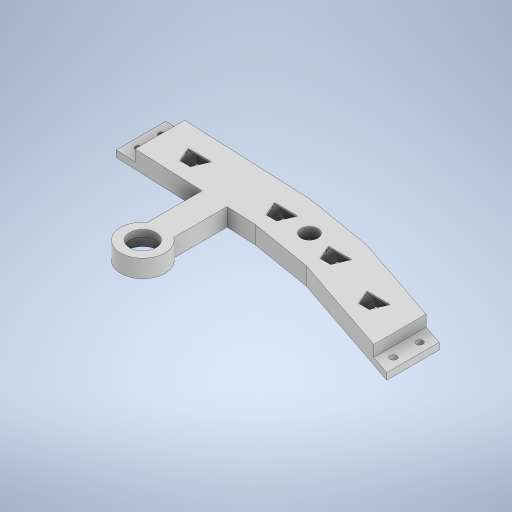
# Autodesk Inventor part: Potentiometer Holder
Saved by Autodesk Inventor 2023 (Build 270158000, 158)
## iProperties
Created: 2022-10-21
Part Number: Potentiometer Holder
Material: Generic
Document SubType Name: Modeling
Designer: GROS
Density: 1 g/cm^3
Appearance: Default
Author: GROS
Autodesk Inventor part; units mm, degrees
ref_plane "YZ Plane" through (0, 0, 0) normal (1, 0, 0) x (0, 1, 0)
ref_plane "XZ Plane" through (0, 0, 0) normal (0, 1, 0) x (-1, 0, 0)
ref_plane "XY Plane" through (0, 0, 0) normal (0, 0, 1) x (1, 0, 0)
sketch "Sketch1" plane through (0, 0, 0) normal (0, 1, 0) x (-1, 0, 0)
  line L0 (104.2041, -28.2127) -> (104.2041, -21.1501)
  line L1 (100.2041, -28.2127) -> (104.2041, -28.2127)
  line L2 (16.1749, -17.7633) -> (10.1749, -17.7633)
  line L3 (10.1749, -17.7633) -> (10.1749, -19.7955)
  line L4 (13.1749, -17.7633) -> (13.1749, -20.8106)
  line L5 (13.1749, -20.8106) -> (13.1749, -4.8696)
  line L6 (13.1749, -20.8106) -> (13.1749, -16.8106)
  line L7 (13.1749, -4.8696) -> (13.1749, -8.8696)
  circle A0 centre (13.1749, -8.8696) radius 1
  circle A1 centre (13.1749, -16.8106) radius 1
  line L8 (10.1749, -19.7955) -> (10.1749, -3.8545)
  circle A2 centre (45.4573, -23.7633) radius 7.55
  line L9 (27.7249, -17.7633) -> (20.1749, -17.7633)
  circle A3 centre (27.7249, -17.7633) radius 7.55
  line L10 (51.451, -33.7618) -> (1.5927, -16.8916)
  line L11 (20.1749, -17.7633) -> (16.1749, -17.7633)
  line L12 (16.1749, -17.7633) -> (16.1749, -5.8847)
  line L13 (16.1749, -17.7633) -> (16.1749, -21.8257)
  circle A4 centre (65.1803, -27.0368) radius 7.55
  line L14 (70.678, -35.6025) -> (39.5208, -30.4313)
  line L15 (107.2041, -28.2127) -> (107.2041, -21.2785)
  line L16 (107.2041, -21.2785) -> (107.2041, -25.2785)
  line L17 (104.2041, -28.2127) -> (104.2041, -36.2639)
  circle A5 centre (107.2041, -32.3923) radius 1
  line L18 (110.2041, -28.2127) -> (110.2041, -21.4069)
  line L19 (107.2041, -28.2127) -> (107.2041, -36.3923)
  line L20 (107.2041, -36.3923) -> (107.2041, -28.3923)
  line L21 (104.2041, -28.2127) -> (110.2041, -28.2127)
  line L22 (110.2041, -28.2127) -> (110.2041, -36.5208)
  circle A6 centre (107.2041, -25.2785) radius 1
  line L23 (114.6217, -21.596) -> (60.8612, -19.295)
  line L24 (60.2143, -34.3811) -> (122.676, -37.0546)
  line L25 (92.6541, -28.2127) -> (100.2041, -28.2127)
  circle A7 centre (92.6541, -28.2127) radius 7.55
  line L26 (51.8932, -17.9704) -> (4.2209, -1.8399)
  line L27 (75.2254, -21.0507) -> (39.3363, -15.0941)
  line L28 (55.3188, -33.0533) -> (55.3188, -17.7467)
  circle A8 centre (55.3188, -25.4) radius 2.55
  circle A9 centre (55.3188, -25.4) radius 1
  line L29 (65.1803, -27.0368) -> (45.4573, -27.0368)
  line L30 (92.6541, -35.7627) -> (92.6541, -28.2127)
  line L31 (65.1803, -34.5868) -> (65.1803, -27.0368)
  line L32 (45.4573, -31.3133) -> (45.4573, -23.7633)
  line L33 (27.7249, -25.3133) -> (27.7249, -17.7633)
  line L34 (92.6541, -28.2127) -> (92.6541, -35.7627)
  line L35 (96.1541, -28.3227) -> (95.1941, -28.3227)
  circle A10 centre (95.1941, -28.3227) radius 0.5
  line L36 (96.1541, -29.3227) -> (93.9142, -23.965)
  line L37 (90.1141, -29.3227) -> (89.1541, -29.3227)
  line L38 (90.1141, -28.3227) -> (90.1141, -29.3227)
  line L39 (89.1541, -29.3227) -> (91.4835, -23.7509)
  circle A11 centre (90.1141, -28.3227) radius 0.5
  line L40 (95.1941, -28.3227) -> (92.6541, -28.3227)
  line L41 (92.6541, -28.3227) -> (92.6541, -25.7827)
  circle A12 centre (92.6541, -25.7827) radius 0.5
  line L42 (92.6541, -28.3227) -> (90.1141, -28.3227)
  line L43 (96.1541, -32.0527) -> (96.1541, -24.8527)
  line L44 (96.1541, -32.0527) -> (96.1541, -28.3227)
  line L45 (96.1541, -24.8527) -> (89.1541, -24.8527)
  line L46 (89.1541, -24.8527) -> (89.1541, -32.0527)
  line L47 (92.6541, -32.0527) -> (96.1541, -32.0527)
  line L48 (89.1541, -29.3227) -> (96.1541, -29.3227)
  line L49 (89.1541, -32.0527) -> (96.1541, -32.0527)
  line L50 (92.6541, -28.2127) -> (92.6541, -32.0527)
  line L51 (92.6541, -35.7627) -> (92.6541, -28.2127)
  line L52 (65.1803, -27.0368) -> (65.1803, -34.5868)
  line L53 (68.6803, -27.1468) -> (67.7203, -27.1468)
  circle A13 centre (67.7203, -27.1468) radius 0.5
  line L54 (68.6803, -28.1468) -> (66.4404, -22.789)
  line L55 (62.6403, -28.1468) -> (61.6803, -28.1468)
  line L56 (62.6403, -27.1468) -> (62.6403, -28.1468)
  line L57 (61.6803, -28.1468) -> (64.0097, -22.5749)
  circle A14 centre (62.6403, -27.1468) radius 0.5
  line L58 (67.7203, -27.1468) -> (65.1803, -27.1468)
  line L59 (65.1803, -27.1468) -> (65.1803, -24.6068)
  circle A15 centre (65.1803, -24.6068) radius 0.5
  line L60 (65.1803, -27.1468) -> (62.6403, -27.1468)
  line L61 (68.6803, -30.8768) -> (68.6803, -23.6768)
  line L62 (68.6803, -30.8768) -> (68.6803, -27.1468)
  line L63 (68.6803, -23.6768) -> (61.6803, -23.6768)
  line L64 (61.6803, -23.6768) -> (61.6803, -30.8768)
  line L65 (65.1803, -30.8768) -> (68.6803, -30.8768)
  line L66 (61.6803, -28.1468) -> (68.6803, -28.1468)
  line L67 (61.6803, -30.8768) -> (68.6803, -30.8768)
  line L68 (65.1803, -27.0368) -> (65.1803, -30.8768)
  line L69 (65.1803, -34.5868) -> (65.1803, -27.0368)
  line L70 (45.4573, -23.7633) -> (45.4573, -31.3133)
  line L71 (48.9573, -23.8733) -> (47.9973, -23.8733)
  circle A16 centre (47.9973, -23.8733) radius 0.5
  line L72 (48.9573, -24.8733) -> (46.7174, -19.5156)
  line L73 (42.9173, -24.8733) -> (41.9573, -24.8733)
  line L74 (42.9173, -23.8733) -> (42.9173, -24.8733)
  line L75 (41.9573, -24.8733) -> (44.2867, -19.3014)
  circle A17 centre (42.9173, -23.8733) radius 0.5
  line L76 (47.9973, -23.8733) -> (45.4573, -23.8733)
  line L77 (45.4573, -23.8733) -> (45.4573, -21.3333)
  circle A18 centre (45.4573, -21.3333) radius 0.5
  line L78 (45.4573, -23.8733) -> (42.9173, -23.8733)
  line L79 (48.9573, -27.6033) -> (48.9573, -20.4033)
  line L80 (48.9573, -27.6033) -> (48.9573, -23.8733)
  line L81 (48.9573, -20.4033) -> (41.9573, -20.4033)
  line L82 (41.9573, -20.4033) -> (41.9573, -27.6033)
  line L83 (45.4573, -27.6033) -> (48.9573, -27.6033)
  line L84 (41.9573, -24.8733) -> (48.9573, -24.8733)
  line L85 (41.9573, -27.6033) -> (48.9573, -27.6033)
  line L86 (45.4573, -23.7633) -> (45.4573, -27.6033)
  line L87 (45.4573, -31.3133) -> (45.4573, -23.7633)
  line L88 (27.7249, -17.7633) -> (27.7249, -25.3133)
  line L89 (31.2249, -17.8733) -> (30.2649, -17.8733)
  circle A19 centre (30.2649, -17.8733) radius 0.5
  line L90 (31.2249, -18.8733) -> (28.985, -13.5156)
  line L91 (25.1849, -18.8733) -> (24.2249, -18.8733)
  line L92 (25.1849, -17.8733) -> (25.1849, -18.8733)
  line L93 (24.2249, -18.8733) -> (26.5542, -13.3014)
  circle A20 centre (25.1849, -17.8733) radius 0.5
  line L94 (30.2649, -17.8733) -> (27.7249, -17.8733)
  line L95 (27.7249, -17.8733) -> (27.7249, -15.3333)
  circle A21 centre (27.7249, -15.3333) radius 0.5
  line L96 (27.7249, -17.8733) -> (25.1849, -17.8733)
  line L97 (31.2249, -21.6033) -> (31.2249, -14.4033)
  line L98 (31.2249, -21.6033) -> (31.2249, -17.8733)
  line L99 (31.2249, -14.4033) -> (24.2249, -14.4033)
  line L100 (24.2249, -14.4033) -> (24.2249, -21.6033)
  line L101 (27.7249, -21.6033) -> (31.2249, -21.6033)
  line L102 (24.2249, -18.8733) -> (31.2249, -18.8733)
  line L103 (24.2249, -21.6033) -> (31.2249, -21.6033)
  line L104 (27.7249, -17.7633) -> (27.7249, -21.6033)
  line L105 (27.7249, -25.3133) -> (27.7249, -17.7633)
  line L106 (92.6541, -28.2127) -> (65.1803, -28.2127)
  line L107 (78.9172, -28.2127) -> (78.9172, 1.7873)
  circle A22 centre (78.9172, 1.7873) radius 4
  circle A23 centre (78.9172, 1.7873) radius 5.25
  circle A24 centre (78.9172, 1.7873) radius 6.75
  line L108 (78.9172, 1.7873) -> (82.9172, 1.7873)
  line L109 (82.9172, 1.7873) -> (74.9172, 1.7873)
  line L110 (74.9172, 1.7873) -> (74.9172, -23.7633)
  line L111 (74.9172, -23.7633) -> (82.9172, -23.7633)
  line L112 (82.9172, -23.7633) -> (82.9172, 1.7873)
  point P0 (47.2973, -16.4154)
  point P1 (43.6173, -31.1112)
  point P2 (64.3979, -34.5602)
  point P3 (65.9627, -19.5133)
  point P4 (24.7236, -17.6804)
  point P5 (26.0936, -14.4033)
  point P6 (29.3561, -14.4033)
  point P7 (30.7262, -17.6804)
  point P8 (30.7649, -17.8733)
  point P9 (30.8068, -17.8733)
  point P10 (24.6889, -17.7633)
  point P11 (24.6971, -17.7633)
  point P12 (43.826, -20.4033)
  point P13 (47.0885, -20.4033)
  point P14 (48.4586, -23.6804)
  point P15 (48.4973, -23.8733)
  point P16 (48.5392, -23.8733)
  point P17 (91.0228, -24.8527)
  point P18 (94.2853, -24.8527)
  point P19 (95.6554, -28.1298)
  point P20 (95.6941, -28.3227)
  point P21 (95.736, -28.3227)
  point P22 (62.179, -26.9539)
  point P23 (63.549, -23.6768)
  point P24 (66.8115, -23.6768)
  point P25 (68.1816, -26.9539)
  point P26 (68.2203, -27.1468)
  point P27 (68.2622, -27.1468)
  point P28 (62.1443, -27.0368)
  point P29 (62.1525, -27.0368)
  point P30 (82.9172, -20.239)
  point P31 (82.9172, -3.6498)
  point P32 (74.9172, -3.6498)
  point P33 (74.9172, -19.8966)
  dimension "d289" = 15.1
  dimension "d369" = 8
  dimension "d282" = 15.1
  dimension "d283" = 15.1
  dimension "d286" = 1.1759
  dimension "d287" = 3.2735
  dimension "d292" = 4
  dimension "d293" = 6
  dimension "d294" = 4
  dimension "d295" = 4
  dimension "d296" = 2
  dimension "d297" = 2
  dimension "d298" = 4
  dimension "d299" = 6
  dimension "d300" = 4
  dimension "d301" = 4
  dimension "d302" = 2
  dimension "d303" = 2
  dimension "d304" = 5.1
  dimension "d305" = 2
  dimension "d307" = 15.1
  dimension "d308" = 7.55
  dimension "d309" = 7.55
  dimension "d310" = 3.84
  dimension "d311" = 3.5
  dimension "d312" = 7.2
  dimension "d313" = 7
  dimension "d314" = 3.73
  dimension "d315" = 0.96
  dimension "d316" = 2.54
  dimension "d317" = 2.54
  dimension "d318" = 2.54
  dimension "d319" = 1
  dimension "d320" = 1
  dimension "d321" = 1
  dimension "d322" = 1
  dimension "d323" = 7.55
  dimension "d324" = 7.55
  dimension "d325" = 3.84
  dimension "d326" = 3.5
  dimension "d327" = 7.2
  dimension "d328" = 7
  dimension "d329" = 3.73
  dimension "d330" = 0.96
  dimension "d331" = 2.54
  dimension "d332" = 2.54
  dimension "d333" = 2.54
  dimension "d334" = 1
  dimension "d335" = 1
  dimension "d336" = 1
  dimension "d337" = 1
  dimension "d338" = 7.55
  dimension "d339" = 7.55
  dimension "d340" = 3.84
  dimension "d341" = 3.5
  dimension "d342" = 7.2
  dimension "d343" = 7
  dimension "d344" = 3.73
  dimension "d345" = 0.96
  dimension "d346" = 2.54
  dimension "d347" = 2.54
  dimension "d348" = 2.54
  dimension "d349" = 1
  dimension "d350" = 1
  dimension "d351" = 1
  dimension "d352" = 1
  constraints: 226 end point, 44 point on line, 23 centre point, 22 coincident, 18 tangent, 11 parallel, 10 vertical, 9 perpendicular, 5 horizontal, 5 midpoint, 2 horizontal alignment, 2 point on circle, 6 other
  measures "d282" diameter of A4
  measures "d283" diameter of A2
  measures "d286" vertical distance of A4.centre A7.centre
  measures "d287" vertical distance of A2.centre A4.centre
  measures "d292" distance of L11.start L13.start
  measures "d293" distance of L13.start L2.end
  measures "d294" distance of L5.end L7.end
  measures "d295" distance of L4.end L6.end
  measures "d296" diameter of A1
  measures "d297" diameter of A0
  measures "d298" distance of L25.end L17.start
  measures "d299" distance of L17.start L21.end
  measures "d300" distance of L15.end L16.end
  measures "d301" distance of point (107.204, -32.392) L19.end
  measures "d302" diameter of A6
  measures "d303" diameter of A5
  measures "d304" diameter of A8
  measures "d305" diameter of A9
  measures "d307" diameter of A7
  measures "d308" distance of L34.start L34.end
  measures "d309" distance of L51.start L50.start
  measures "d310" distance of L50.start L47.start
  measures "d311" distance of L47.start L47.end
  measures "d312" distance of L47.end L43.end
  measures "d313" distance of L46.end L47.end
  measures "d314" distance of L47.end L35.start
  measures "d315" distance of L35.start L40.start
  measures "d316" distance of L40.start L40.end
  measures "d317" distance of L40.end L42.end
  measures "d318" distance of L40.end L41.end
  measures "d319" diameter of A12
  measures "d320" diameter of A10
  measures "d321" diameter of A11
  measures "d322" distance of L38.start L37.start
  measures "d323" distance of L52.start L52.end
  measures "d324" distance of L69.start L68.start
  measures "d325" distance of L68.start L65.start
  measures "d326" distance of L65.start L65.end
  measures "d327" distance of L65.end L61.end
  measures "d328" distance of L64.end L65.end
  measures "d329" distance of L65.end L53.start
  measures "d330" distance of L53.start L58.start
  measures "d331" distance of L58.start L58.end
  measures "d332" distance of L58.end L60.end
  measures "d333" distance of L58.end L59.end
  measures "d334" diameter of A15
  measures "d335" diameter of A13
  measures "d336" diameter of A14
  measures "d337" distance of L56.start L55.start
  measures "d338" distance of L70.start L70.end
  measures "d339" distance of L87.start L86.start
  measures "d340" distance of L86.start L83.start
  measures "d341" distance of L83.start L83.end
  measures "d342" distance of L83.end L79.end
  measures "d343" distance of L82.end L83.end
  measures "d344" distance of L83.end L71.start
  measures "d345" distance of L71.start L76.start
  measures "d346" distance of L76.start L76.end
  measures "d347" distance of L76.end L78.end
  measures "d348" distance of L76.end L77.end
  measures "d349" diameter of A18
  measures "d350" diameter of A16
  measures "d351" diameter of A17
  measures "d352" distance of L74.start L73.start
extrude "Extrusion1" add sketch "Sketch1" against normal blind 4.9 contours L1 A7 L23 L0 | L17 L24 A7 L1 | A7 L30 L47 L43 L25 | L25 L43 L45 L46 L106 A7 | A7 L106 L107 L111 L112 L23 | A7 L106 L46 L49 L30 | L24 A4 L106 A7 | L112 L111 L107 L23 | L24 L14 A4 | A4 L29 L64 L67 L31 | L107 L111 L110 L23 | L106 A4 L27 L110 L111 L107 | L14 L28 A8 L29 A4 | L31 L65 L61 L106 A4 | L110 L27 L23 | L106 L61 L63 L64 L29 A4 A8 | L29 A8 A4 | L14 A2 L29 A8 L28 | L27 A4 L23 | L23 A4 A8 L28 L27 | A8 L29 L28 A9 A4 | A4 A8 | A8 L28 L29 | L14 L10 A2 | A2 A8 L29 L79 L81 L82 L85 L32 | A8 L29 L28 | L28 A8 A2 L26 L27 | L29 A8 A2 L28 A9 | L10 A3 L26 L27 A2 | L32 L83 L79 L29 A2 | L29 A2 A8 | L26 A2 L27 | A9 L28 | L28 A9 | L10 L13 L11 A3 | A3 L9 L100 L103 L33 | A8 A2 | A3 L33 L101 L97 L99 L100 L9 | A3 L11 L12 L26
extrude "Extrusion2" add sketch "Sketch1" along normal blind 0.5 contours L1 A7 L23 L0 | L17 L24 A7 L1 | A7 L30 L47 L43 L25 | L25 L43 L45 L46 L106 A7 | A7 L106 L107 L111 L112 L23 | L43 L35 L36 L25 | L25 L36 L45 L43 | A7 L106 L46 L49 L30 | L24 A4 L106 A7 | L112 L111 L107 L23 | L36 L35 A10 L25 | L25 A10 L36 | L43 L36 L35 | L49 L46 L37 L48 L30 | L30 L48 L43 L47 | L24 L14 A4 | A4 L29 L64 L67 L31 | L107 L111 L110 L23 | L106 L39 L46 | L46 L45 L39 L106 | L106 A4 L27 L110 L111 L107 | L14 L28 A8 L29 A4 | L31 L65 L61 L106 A4 | L110 L27 L23 | L106 L61 L63 L64 L29 A4 A8 | L29 A8 A4 | L14 A2 L29 A8 L28 | L67 L64 L55 L66 L31 | L31 L106 L61 L65 | L27 A4 L23 | L23 A4 A8 L28 L27 | L106 L31 L66 L61 | A8 L29 L28 A9 A4 | A4 A8 | L64 L63 L57 L29 | L29 L57 L64 | A8 L28 L29 | L14 L10 A2 | A2 A8 L29 L79 L81 L82 L85 L32 | A8 L29 L28 | L28 A8 A2 L26 L27 | L54 L53 L61 | L57 A14 L29 | L29 A8 A2 L28 A9 | L10 A3 L26 L27 A2 | L32 L83 L79 L29 A2 | L29 A2 A8 | L26 A2 L27 | L54 L63 L61 L53 | L53 A13 L54 | A9 L28 | L28 A9 | L10 L13 L11 A3 | A3 L9 L100 L103 L33 | L85 L82 L73 L84 L32 | L32 L29 L79 L83 | A8 A2 | A3 L33 L101 L97 L99 L100 L9 | A3 L11 L12 L26 | L29 L32 L84 L79 | L100 L99 L93 L9 | L9 L93 L100 | L103 L100 L91 L102 L33 | L33 L102 L97 L101 | L72 L71 L79 | L82 L81 L75 | L93 A20 L9 | L72 L81 L79 L71 | L71 A16 L72 | L90 L89 L97 | L99 L97 L89 L90 | L89 A19 L90
extrude "Extrusion4" add sketch "Sketch1" against normal up to surface (4.9 mm away) contours L21 L19 A5 L24 L17 | L0 L23 L15 A6 L21 | L21 L22 L24 L19 A5 | L15 A6 L23 L18 L21 | L10 L4 A1 L2 L13 | L12 L2 A1 L5 A0 L26 | L10 L3 L2 A1 L4 | L5 A0 A1 L2 L8 L26
extrude "Extrusion5" cut sketch "Sketch1" against normal blind 2.9 contours L21 L19 A5 L24 L17 | L0 L23 L15 A6 L21 | L21 L22 L24 L19 A5 | L15 A6 L23 L18 L21 | L10 L4 A1 L2 L13 | L12 L2 A1 L5 A0 L26 | L10 L3 L2 A1 L4 | L5 A0 A1 L2 L8 L26
extrude "Extrusion6" cut sketch "Sketch1" along normal blind 0.5 and the other way blind 2.9 contours A8 L29 L28 A9 A4 | A4 A8 | A8 L28 L29 | A8 L29 L28 | L29 A8 A2 L28 A9 | A9 L28 | L28 A9 | A8 A2
extrude "Extrusion7" cut sketch "Sketch1" against normal up to surface (4.9 mm away) contours A9 L28 | L28 A9
extrude "Extrusion8" add sketch "Sketch1" along normal blind 0.5 and the other way blind 4.9 contours L23 L107 A24 L112 | L23 L110 A24 L107 | L112 A23 L110 A24 | A24 L107 A23 L112 | A24 L110 A23 L107
extrude "Extrusion9" add sketch "Sketch1" along normal blind 0.5 and the other way blind 1.5 contours L112 A22 L110 A23 | A23 L107 A22 L112 | A23 L110 A22 L107
body "Solid1"
